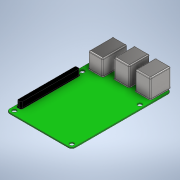
# Autodesk Inventor part: RPi Subs
Saved by Autodesk Inventor 2020.1 (Build 241239000, 239)
## iProperties
Created: 2022-03-19
Part Number: RPi Subs
Material: Generic
Document SubType Name: Modeling
Designer: OEM
Density: 1 g/cm^3
Appearance: Default
Author: OEM
Autodesk Inventor part; units mm, degrees
ref_plane "YZ Plane" through (0, 0, 0) normal (1, 0, 0) x (0, 1, 0)
ref_plane "XZ Plane" through (0, 0, 0) normal (0, 1, 0) x (-1, 0, 0)
ref_plane "XY Plane" through (0, 0, 0) normal (0, 0, 1) x (1, 0, 0)
sketch "Sketch1" plane through (0, 0, 0) normal (0, 1, 0) x (-1, 0, 0)
  line L0 (28, 42.5) -> (-28, 42.5)
  line L1 (-28, 42.5) -> (-28, -42.5)
  line L2 (-28, -42.5) -> (28, -42.5)
  line L3 (28, -42.5) -> (28, 42.5)
  line L4 (28, 42.5) -> (-28, -42.5) construction
  line L5 (-28, 42.5) -> (28, -42.5) construction
  circle A0 centre (-24.5, 39) radius 1.75
  line L6 (35, 10) -> (-43, 10) construction
  circle A1 centre (-24.5, -19) radius 1.75
  line L7 (0, 50) -> (0, -62) construction
  circle A2 centre (24.5, 39) radius 1.75
  circle A3 centre (24.5, -19) radius 1.75
  line L8 (-19, -42.5) -> (-19, -27) construction
  line L9 (-1, -42.5) -> (-1, -27) construction
  line L10 (17.75, -42.5) -> (17.75, -27) construction
  line L11 (-25.5, -42.5) -> (-25.5, -27)
  line L12 (-25.5, -27) -> (-19, -27)
  line L13 (-25.5, -42.5) -> (-25.5, -44.5)
  line L14 (-25.5, -44.5) -> (-20, -44.5)
  line L15 (-12.5, -42.5) -> (-12.5, -27)
  line L16 (-12.5, -27) -> (-19, -27)
  line L17 (-12.5, -42.5) -> (-12.5, -44.5)
  line L18 (-12.5, -44.5) -> (-20, -44.5)
  line L19 (-1, -27) -> (-7.5, -27)
  line L20 (-7.5, -27) -> (-7.5, -44.5)
  line L21 (-7.5, -44.5) -> (-1, -44.5)
  line L22 (-1, -27) -> (5.5, -27)
  line L23 (5.5, -27) -> (5.5, -44.5)
  line L24 (5.5, -44.5) -> (-1, -44.5)
  line L25 (17.75, -23.5) -> (11.6404, -23.5)
  line L26 (11.6404, -23.5) -> (11.6404, -44.5)
  line L27 (11.6404, -44.5) -> (17.75, -44.5)
  line L28 (17.75, -23.5) -> (23.8596, -23.5)
  line L29 (23.8596, -23.5) -> (23.8596, -44.5)
  line L30 (23.8596, -44.5) -> (17.75, -44.5)
  line L31 (24.5, 39) -> (24.5, -19) construction
  line L32 (24.5, 35) -> (26.25, 35)
  line L33 (26.25, 35) -> (26.25, 10)
  line L34 (24.5, 35) -> (22.75, 35)
  line L35 (22.75, 35) -> (22.75, 10)
  line L36 (24.5, -15) -> (26.25, -15)
  line L37 (26.25, -15) -> (26.25, 10)
  line L38 (22.75, -15) -> (22.75, 10)
  line L39 (24.5, -15) -> (22.75, -15)
  point P0 (0, 0)
  point P1 (0, 0)
  point P2 (-7.5, -42.5)
  point P3 (5.5, -42.5)
  point P4 (11.6404, -42.5)
  point P5 (23.8596, -42.5)
  dimension "d0" = 56
  dimension "d1" = 85
  dimension "d2" = 3.5
  dimension "d3" = 3.5
  dimension "d4" = 3.5
  dimension "d5" = 29
  dimension "d6" = 49
  dimension "d7" = 58
  dimension "d11" = 9
  dimension "d12" = 27
  dimension "d13" = 45.75
  dimension "d14" = 2
  dimension "d15" = 6.5
  dimension "d18" = 6.5
  dimension "d19" = 21
  constraints: 80 end point, 15 symmetric about line, 9 perpendicular, 7 point on line, 6 horizontal, 5 vertical, 4 centre point, 3 midpoint, 2 parallel, 3 other
  measures "d0" distance of L2.end L1.end
  measures "d1" distance of L1.end L0.end
  measures "d2" diameter of A0
  measures "d3" distance from line of L0 A0.centre
  measures "d4" distance from line of L1 A0.centre
  measures "d5" distance from line of L6 A0.centre
  measures "d6" distance of A0.centre L31.start
  measures "d7" distance of A0.centre A1.centre
  measures "d11" distance between parallel lines of L1 L8
  measures "d12" distance between parallel lines of L9 L1
  measures "d13" distance between parallel lines of L10 L1
  measures "d14" distance of L11.start L13.end
  measures "d15" distance between parallel lines of L11 L8
  measures "d18" distance of L9.end L19.end
  measures "d19" distance of L25.end L26.end
extrude "Extrusion1" add sketch "Sketch1" against normal blind 1 contours L3 L2 L29 L28 L25 L26 L23 L22 L19 L20 L15 L16 L12 L11 L1 L0 | L2 L26 L25 L28 L29 | L11 L12 L16 L15 L2 | L2 L20 L19 L22 L23 | L32 L33 L37 L36 L39 L38 L35 L34
fillet "Fillet1" radius 3 4 edges at (28, -0.5, 42.5) (-28, -0.5, 42.5) (-28, -0.5, -42.5) (28, -0.5, -42.5)
extrude "Extrusion2" add sketch "Sketch1" along normal blind 16 contours L11 L12 L16 L15 L2 | L2 L17 L18 L14 L13 | L23 L24 L21 L20 L2 | L2 L20 L19 L22 L23
extrude "Extrusion3" add sketch "Sketch1" along normal blind 13.5 contours L29 L30 L27 L26 L2 | L2 L26 L25 L28 L29
fillet "Fillet2" radius 1 27 edges at (25.5, 16, -35.75) (19, 16, -44.5) (25.5, 8, -44.5) (25.5, 8, -27) (19, 16, -27) (12.5, 8, -27) (12.5, 16, -35.75) (12.5, 8, -44.5) (-5.5, 8, -44.5) (1, 16, -44.5) (7.5, 8, -44.5) (-5.5, 16, -35.75) (7.5, 16, -35.75) (1, 16, -27) (-5.5, 8, -27) (7.5, 8, -27) (-11.6404, 6.75, -23.5) (-17.75, 13.5, -23.5) (-23.8596, 6.75, -23.5) (-23.8596, 13.5, -34) (-17.75, 13.5, -44.5) (-11.6404, 6.75, -44.5) (-23.8596, 6.75, -44.5) (-11.6404, 13.5, -34) (19, 0, -44.5) (1, 0, -44.5) (-17.75, 0, -44.5)
extrude "Extrusion4" add sketch "Sketch1" along normal blind 5 contours L32 L33 L37 L36 L39 L38 L35 L34
fillet "Fillet3" radius 1 4 edges at (-22.75, 2.5, 35) (-26.25, 2.5, 35) (-22.75, 2.5, -15) (-26.25, 2.5, -15)
fillet "Fillet4" radius 0.5 23 edges at (-23.0429, 0, 34.7071) (-24.5, 0, 35) (-25.9571, 0, 34.7071) (-26.25, 0, 10) (-25.9571, 0, -14.7071) (-24.5, 0, -15) (-23.0429, 0, -14.7071) (-22.75, 0, 10) (25.2071, 0, -27.2929) (19, 0, -27) (12.7929, 0, -27.2929) (12.5, 0, -35.25) (25.5, 0, -35.229) (-11.6404, 0, -33.5) (-17.75, 0, -23.5) (-23.5667, 0, -23.7929) (-23.8596, 0, -33.5) (-11.9333, 0, -23.7929) (-5.2071, 0, -27.2929) (-5.5, 0, -35.25) (7.2071, 0, -27.2929) (7.5, 0, -35.25) (1, 0, -27)
fillet "Fillet5" radius 0.1 18 edges at (27.4495, 0, -41.2321) (25.6415, 0.1514, -42.4306) (27.1213, 0, 41.6213) (0, 0, 42.5) (-27.1213, 0, 41.6213) (-28, 0, 0) (-27.1213, 0, -41.6213) (-24.6798, 0, -42.5) (-24.006, 0.1464, -42.5) (28, 0, 0) (27.1213, -1, 41.6213) (0, -1, 42.5) (-27.1213, -1, 41.6213) (-28, -1, 0) (-27.1213, -1, -41.6213) (0, -1, -42.5) (27.1213, -1, -41.6213) (28, -1, 0)
body "Solid1"
